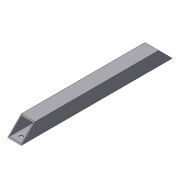
# Autodesk Inventor part: Frame_LowerCrossSupport
Saved by Autodesk Inventor 2012 (Build 160160000, 160)
## iProperties
Created: 2012-01-14
Part Number: Frame_LowerCrossSupport
Material: Aluminum-6061
Document SubType Name: Modeling
Designer: JesseK
Mass: 103.799 g
Surface Area: 487.551 cm^2
Volume: 38.3021 cm^3
Density: 2.71 g/cm^3
Author: JesseK
Autodesk Inventor part; units mm, degrees
ref_plane "YZ Plane" through (0, 0, 0) normal (1, 0, 0) x (0, 1, 0)
ref_plane "XZ Plane" through (0, 0, 0) normal (0, 1, 0) x (-1, 0, 0)
ref_plane "XY Plane" through (0, 0, 0) normal (0, 0, 1) x (1, 0, 0)
sketch "Sketch1" plane through (0, 0, 0) normal (0, 0, 1) x (1, 0, 0)
  line L0 (0, 0) -> (25.4, 0)
  line L1 (25.4, 0) -> (25.4, 25.4)
  line L2 (25.4, 25.4) -> (0, 25.4)
  line L3 (0, 25.4) -> (0, 0)
  dimension "d0" = 25.4
  dimension "d1" = 25.4
  constraints: 8 end point, 2 parallel, 1 horizontal, 1 perpendicular
  measures "d0" distance of L1.end L2.end
  measures "d1" distance of L0.end L1.end
extrude "Extrusion1" add sketch "Sketch1" along normal blind 279.4
shell "Shell1" thickness 1.5875 removed faces 2 at (8.4667, 16.9333, 0) at (8.4667, 16.9333, 279.4)
sketch "Sketch2" plane through (25.4, 0, 0) normal (1, 0, 0) x (0, 0, -1)
  line L0 (-279.4, 25.4) -> (-279.4, 0) projected
  line L1 (0, 0) -> (0, 25.4) projected
  line L2 (0, 25.4) -> (-279.4, 25.4) projected
  line L3 (-279.4, 0) -> (-279.4, 25.4)
  line L4 (-254, 25.4) -> (-279.4, 25.4)
  line L5 (-279.4, 0) -> (-254, 25.4)
  line L6 (0, 25.4) -> (0, 0)
  line L7 (-25.4, 25.4) -> (0, 0)
  line L8 (-25.4, 25.4) -> (0, 25.4)
  dimension "d5" = 25.4
  dimension "d6" = 25.4
  constraints: 12 end point, 2 horizontal, 2 point on line, 2 vertical
  measures "d5" distance of L0.start L4.start
  measures "d6" distance of L1.end L7.start
extrude "Extrusion2" cut sketch "Sketch2" against normal through all
sketch "Sketch3" plane through (0, 0, 279.4) normal (0, -1, 0) x (1, 0, 0)
  line L0 (25.4, 0) -> (0, 0) projected
  line L1 (0, -279.4) -> (25.4, -279.4) projected
  line L2 (25.4, -279.4) -> (25.4, 0) projected
  circle A0 centre (12.7, -12.7) radius 3.175
  circle A1 centre (12.7, -266.7) radius 3.175
  dimension "d9" = 6.35
  dimension "d10" = 12.7
  dimension "d11" = 12.7
  dimension "d12" = 12.7
  dimension "d13" = 12.7
  constraints: 2 centre point, 1 equal radius
  measures "d9" diameter of A0
  measures "d10" distance from line of L2 A0.centre
  measures "d11" distance from line of L0 A0.centre
  measures "d12" distance from line of L2 A1.centre
  measures "d13" distance from line of L1 A1.centre
extrude "Extrusion3" cut sketch "Sketch3" against normal through all
sketch "Sketch4" plane through (25.4, 0, 279.4) normal (1, 0, 0) x (0, 0, -1)
  circle A0 centre (20.2966, 9.5234) radius 0.9528
  constraints: 1 centre point
extrude "Extrusion4" cut sketch "Sketch4" against normal up to next
body "Solid1"
